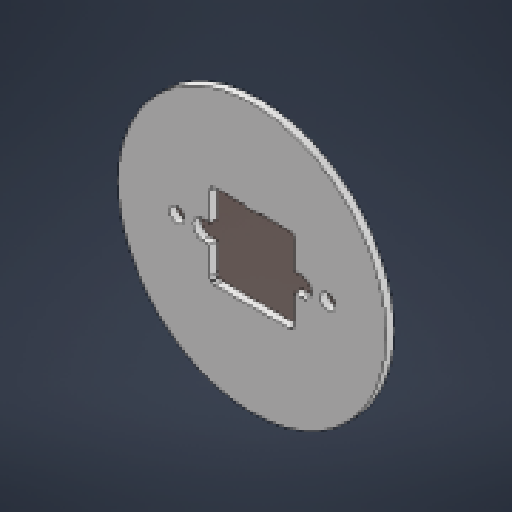
# Autodesk Inventor part: Mirror_Hub
Saved by Autodesk Inventor 2024.2 (Build 282272000, 272)
## iProperties
Created: 2023-12-27
Part Number: Mirror_Hub
Material: 一般
Document SubType Name: Modeling
Designer: Hanaoka
Density: 1 g/cm^3
Appearance: 既定
Author: Hanaoka
Autodesk Inventor part; units mm, degrees
ref_plane "YZ Plane" through (0, 0, 0) normal (1, 0, 0) x (0, 1, 0)
ref_plane "XZ Plane" through (0, 0, 0) normal (0, 1, 0) x (-1, 0, 0)
ref_plane "XY Plane" through (0, 0, 0) normal (0, 0, 1) x (1, 0, 0)
ref_plane "作業平面1" through (0, 0, 0) normal (0, 0, 1) x (1, 0, 0)
sketch "スケッチ1" plane through (0, 0, 0) normal (0, 0, 1) x (1, 0, 0)
  line L0 (16.51, 16.51) -> (0, 16.51) projected
  line L1 (0, 16.51) -> (0, 11.176) projected
  line L2 (0, 11.176) -> (-6.731, 11.176) projected
  line L3 (-6.731, 11.176) -> (-7.4684, 11.0622) projected
  line L4 (-7.4684, 11.0622) -> (-8.1512, 10.7614) projected
  line L5 (-8.1512, 10.7614) -> (-8.733, 10.2942) projected
  line L6 (-8.733, 10.2942) -> (-9.1739, 9.6923) projected
  line L7 (-9.1739, 9.6923) -> (-9.4441, 8.9967) projected
  line L8 (-9.4441, 8.9967) -> (-9.525, 8.255) projected
  line L9 (-9.525, 8.255) -> (-9.4441, 7.5133) projected
  line L10 (-9.4441, 7.5133) -> (-9.1739, 6.8177) projected
  line L11 (-9.1739, 6.8177) -> (-8.733, 6.2158) projected
  line L12 (-8.733, 6.2158) -> (-8.1512, 5.7486) projected
  line L13 (-8.1512, 5.7486) -> (-7.4684, 5.4478) projected
  line L14 (-7.4684, 5.4478) -> (-6.731, 5.334) projected
  line L15 (-6.731, 5.334) -> (0, 5.334) projected
  line L16 (0, 5.334) -> (0, 0) projected
  line L17 (0, 0) -> (16.51, 0) projected
  line L18 (16.51, 0) -> (16.51, 5.334) projected
  line L19 (16.51, 5.334) -> (23.241, 5.334) projected
  line L20 (23.241, 5.334) -> (23.9784, 5.4478) projected
  line L21 (23.9784, 5.4478) -> (24.6612, 5.7486) projected
  line L22 (24.6612, 5.7486) -> (25.243, 6.2158) projected
  line L23 (25.243, 6.2158) -> (25.6839, 6.8177) projected
  line L24 (25.6839, 6.8177) -> (25.9541, 7.5133) projected
  line L25 (25.9541, 7.5133) -> (26.035, 8.255) projected
  line L26 (26.035, 8.255) -> (25.9541, 8.9967) projected
  line L27 (25.9541, 8.9967) -> (25.6839, 9.6923) projected
  line L28 (25.6839, 9.6923) -> (25.243, 10.2942) projected
  line L29 (25.243, 10.2942) -> (24.6612, 10.7614) projected
  line L30 (24.6612, 10.7614) -> (23.9784, 11.0622) projected
  line L31 (23.9784, 11.0622) -> (23.241, 11.176) projected
  line L32 (23.241, 11.176) -> (16.51, 11.176) projected
  line L33 (16.51, 11.176) -> (16.51, 16.51) projected
  circle A0 centre (18.26, 8.26) radius 1.27 projected
  circle A1 centre (-1.75, 8.26) radius 1.27 projected
  circle A2 centre (11.505, 9.45) radius 0.127 projected
  circle A3 centre (8.386, 9.267) radius 0.127 projected
  circle A4 centre (4.826, 15.748) radius 0.127 projected
  circle A5 centre (4.191, 15.748) radius 0.127 projected
  circle A6 centre (-6.985, 8.255) radius 1.5 projected
  circle A7 centre (23.495, 8.255) radius 1.5 projected
  circle A8 centre (3.048, 4.445) radius 0.1651 projected
  circle A9 centre (6.985, 4.445) radius 0.1651 projected
  circle A10 centre (2.286, 6.731) radius 0.2032 projected
  circle A11 centre (13.716, 8.509) radius 0.2032 projected
  circle A12 centre (12.319, 1.778) radius 0.2032 projected
  circle A13 centre (15.367, 16.002) radius 0.2032 projected
  circle A14 centre (14.732, 1.778) radius 0.2032 projected
  circle A15 centre (13.462, 1.778) radius 0.2032 projected
  circle A16 centre (11.5062, 15.748) radius 0.127 projected
  circle A17 centre (7.874, 15.748) radius 0.127 projected
  circle A18 centre (3.429, 14.859) radius 0.127 projected
  circle A19 centre (14.478, 15.113) radius 0.1651 projected
  circle A20 centre (2.286, 10.541) radius 0.2032 projected
  circle A21 centre (13.716, 11.176) radius 0.2032 projected
  circle A22 centre (5.505, 15.748) radius 0.127 projected
  circle A23 centre (14.478, 14.224) radius 0.1651 projected
  circle A24 centre (13.462, 15.113) radius 0.1651 projected
  circle A25 centre (10.414, 15.7988) radius 0.127 projected
  circle A26 centre (5.005, 9.727) radius 0.127 projected
  circle A27 centre (6.8072, 8.636) radius 0.127 projected
  circle A28 centre (4.699, 8.382) radius 0.127 projected
  circle A29 centre (10.922, 8.636) radius 0.127 projected
  circle A30 centre (6.378, 16.129) radius 0.127 projected
  circle A31 centre (10.4648, 5.4864) radius 0.127 projected
  circle A32 centre (11.2268, 5.4864) radius 0.127 projected
  circle A33 centre (10.4648, 6.1214) radius 0.127 projected
  circle A34 centre (9.1948, 7.8994) radius 0.127 projected
  circle A35 centre (2.955, 14.2) radius 0.3 projected
  circle A36 centre (9.779, 15.748) radius 0.127 projected
  circle A37 centre (9.906, 8.636) radius 0.127 projected
  circle A38 centre (9.194, 7.112) radius 0.127 projected
  circle A39 centre (9.144, 15.748) radius 0.127 projected
  circle A40 centre (5.588, 7.874) radius 0.127 projected
  circle A41 centre (13.335, 6.096) radius 0.1651 projected
  circle A42 centre (6.8072, 7.874) radius 0.127 projected
  circle A43 centre (6.878, 15.748) radius 0.127 projected
  circle A44 centre (7.378, 16.141) radius 0.127 projected
  circle A45 centre (5.588, 7.239) radius 0.127 projected
  circle A46 centre (8.509, 15.748) radius 0.127 projected
  circle A47 centre (7.5946, 7.1186) radius 0.127 projected
  circle A48 centre (13.555, 14.2) radius 0.3 projected
  line L34 (9.655, 16.755) -> (9.655, 15.8775) projected
  arc A49 (6.855, 15.8775) -> (9.655, 15.8775) centre (8.255, 8.255) ccw projected
  line L35 (6.855, 15.8775) -> (6.855, 16.755) projected
  line L36 (6.855, 16.755) -> (0.755, 16.755) projected
  arc A50 (0.755, 16.755) -> (-0.245, 15.755) centre (0.755, 15.755) ccw projected
  line L37 (-0.245, 15.755) -> (-0.245, 10.155) projected
  line L38 (-0.245, 10.155) -> (-1.745, 10.155) projected
  arc A51 (-1.745, 10.155) -> (-1.745, 6.355) centre (-1.745, 8.255) ccw projected
  line L39 (-1.745, 6.355) -> (-0.245, 6.355) projected
  line L40 (-0.245, 6.355) -> (-0.245, 0.755) projected
  arc A52 (-0.245, 0.755) -> (0.755, -0.245) centre (0.755, 0.755) ccw projected
  line L41 (0.755, -0.245) -> (15.755, -0.245) projected
  arc A53 (15.755, -0.245) -> (16.755, 0.755) centre (15.755, 0.755) ccw projected
  line L42 (16.755, 0.755) -> (16.755, 6.355) projected
  line L43 (16.755, 6.355) -> (18.255, 6.355) projected
  arc A54 (18.255, 6.355) -> (18.255, 10.155) centre (18.255, 8.255) ccw projected
  line L44 (18.255, 10.155) -> (16.755, 10.155) projected
  line L45 (16.755, 10.155) -> (16.755, 15.755) projected
  arc A55 (16.755, 15.755) -> (15.755, 16.755) centre (15.755, 15.755) ccw projected
  line L46 (15.755, 16.755) -> (9.655, 16.755) projected
  circle A56 centre (-1.745, 8.255) radius 0.9 projected
  circle A57 centre (18.255, 8.255) radius 0.9 projected
  circle A58 centre (8.255, 8.255) radius 27
  point P0 (0, 16.4107)
  point P1 (0.0993, 16.51)
  point P2 (6.855, 16.51)
  point P3 (9.655, 16.51)
  point P4 (16.4107, 16.51)
  point P5 (16.51, 16.4107)
  point P6 (16.51, 0.0993)
  point P7 (16.4107, 0)
  point P8 (0.0993, 0)
  point P9 (0, 0.0993)
  dimension "d0" = 54
  constraints: 1 centre point, 1 coincident
  measures "d0" diameter of A58
extrude "押し出し1" add sketch "スケッチ1" along normal blind 1.5 contours L32 L31 L30 L29 L28 L27 L26 L25 L24 L23 L22 L21 L20 L19 L42 L43 A54 L44 L45 | L37 L38 A51 L39 L40 L15 L14 L13 L12 L11 L10 L9 L8 L7 L6 L5 L4 L3 L2 | A58
